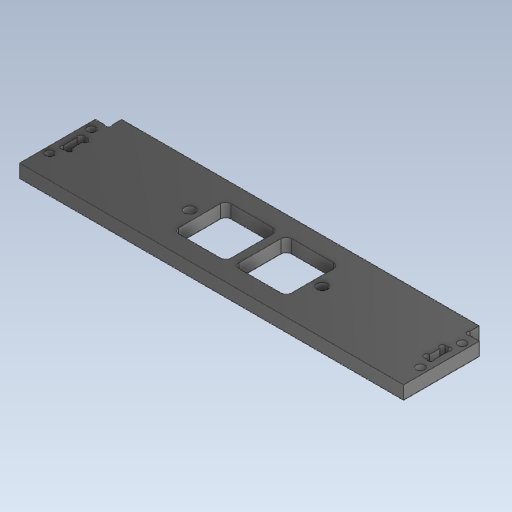
# Autodesk Inventor part: Cockpit_top_frame
Saved by Autodesk Inventor 2020.4 (Build 244396000, 396)
## iProperties
Created: 2022-01-28
Part Number: Cockpit_top_frame
Material: アセタール樹脂、黒
Document SubType Name: Modeling
Designer: Masato Kubotera
Density: 1.425 g/cm^3
Appearance: 滑らか - 黒
Description: POM T5
Author: Masato Kubotera
Autodesk Inventor part; units mm, degrees
ref_plane "YZ Plane" through (0, 0, 0) normal (1, 0, 0) x (0, 1, 0)
ref_plane "XZ Plane" through (0, 0, 0) normal (0, 1, 0) x (-1, 0, 0)
derived "Cockpit_side_frame.ipt"
sketch "スケッチ2" plane through (0, 0, 0) normal (0, 1, 0) x (-1, 0, 0)
  line L0 (-28.5, -22.5) -> (88.5, -22.5) construction
  line L1 (88.5, -22.5) -> (88.5, -138.5)
  line L2 (88.5, -96) -> (-28.5, -96) construction
  line L3 (-28.5, -96) -> (-28.5, -22.5) construction
  line L4 (-28.5, -22.5) -> (88.5, -96) construction
  line L5 (88.5, -22.5) -> (-28.5, -96) construction
  line L6 (38.5, -101) -> (38.5, -133.5)
  line L7 (43.5, -138.5) -> (88.5, -138.5)
  arc A0 (64.6349, -63.15) -> (63.15, -64.6349) centre (63.8925, -63.8925) ccw
  arc A1 (73.15, -65.2849) -> (71.6651, -63.8) centre (72.4075, -64.5425) ccw
  line L8 (65.3349, -63.8) -> (71.6651, -63.8)
  line L9 (64.6349, -63.15) -> (72.3651, -63.15)
  line L10 (63.9, -63.85) -> (73.1, -63.85) construction
  arc A2 (65.3349, -63.8) -> (63.85, -65.2849) centre (64.5925, -64.5425) ccw
  line L11 (63.2, -63.2) -> (73.8, -63.2) construction
  line L12 (73.15, -65.2849) -> (73.15, -76.2151)
  line L13 (73.8, -70.75) -> (63.2, -70.75) construction
  line L14 (73.85, -64.6349) -> (73.85, -76.8651)
  line L15 (73.1, -63.85) -> (73.1, -77.65) construction
  line L16 (63.85, -65.2849) -> (63.85, -76.2151)
  line L17 (73.8, -63.2) -> (73.8, -78.3) construction
  line L18 (63.15, -64.6349) -> (63.15, -76.8651)
  line L19 (68.5, -63.2) -> (68.5, -78.3) construction
  line L20 (63.9, -77.65) -> (63.9, -63.85) construction
  line L21 (73.1, -63.85) -> (63.9, -77.65) construction
  line L22 (73.8, -63.2) -> (63.2, -78.3) construction
  line L23 (63.2, -63.2) -> (73.8, -78.3) construction
  line L24 (63.2, -78.3) -> (63.2, -63.2) construction
  line L25 (63.9, -63.85) -> (73.1, -77.65) construction
  arc A3 (73.85, -64.6349) -> (72.3651, -63.15) centre (73.1075, -63.8925) ccw
  line L26 (73.1, -77.65) -> (63.9, -77.65) construction
  line L27 (73.8, -78.3) -> (63.2, -78.3) construction
  arc A4 (63.85, -76.2151) -> (65.3349, -77.7) centre (64.5925, -76.9575) ccw
  arc A5 (63.15, -76.8651) -> (64.6349, -78.35) centre (63.8925, -77.6075) ccw
  line L28 (65.3349, -77.7) -> (71.6651, -77.7)
  line L29 (64.6349, -78.35) -> (72.3651, -78.35)
  arc A6 (71.6651, -77.7) -> (73.15, -76.2151) centre (72.4075, -76.9575) ccw
  arc A7 (72.3651, -78.35) -> (73.85, -76.8651) centre (73.1075, -77.6075) ccw
  line L30 (-23.5, -22.5) -> (-28.5, -27.5)
  line L31 (-28.5, -59.25) -> (88.5, -59.25) construction
  line L32 (30, -22.5) -> (30, -96) construction
  line L33 (-23.5, -96) -> (-28.5, -91)
  line L34 (-28.5, -27.5) -> (-28.5, -91)
  line L35 (-20.5, -24.5) -> (-25.5, -24.5) construction
  line L36 (-25.5, -24.5) -> (-25.5, -94) construction
  line L37 (-25.5, -94) -> (-20.5, -94) construction
  line L38 (-20.5, -94) -> (-20.5, -24.5) construction
  line L39 (-20.5, -24.5) -> (-25.5, -94) construction
  line L40 (-25.5, -24.5) -> (-20.5, -94) construction
  line L41 (-25.55, -46.7) -> (-20.45, -46.7)
  line L42 (-20.45, -46.7) -> (-20.45, -71.8)
  line L43 (-20.45, -71.8) -> (-25.55, -71.8)
  line L44 (-25.55, -71.8) -> (-25.55, -46.7)
  line L45 (-25.55, -46.7) -> (-20.45, -71.8) construction
  line L46 (-20.45, -46.7) -> (-25.55, -71.8) construction
  line L47 (-25.5, -46.75) -> (-20.5, -46.75) construction
  line L48 (-25.5, -71.75) -> (-20.5, -71.75) construction
  line L49 (-23, -24.5) -> (-23, -94) construction
  circle A8 centre (-23, -35) radius 3
  circle A9 centre (-23, -35) radius 1.6
  arc A10 (-24.0651, -46.7) -> (-25.55, -48.1849) centre (-24.8075, -47.4425) ccw
  arc A11 (-20.45, -48.1849) -> (-21.9349, -46.7) centre (-21.1925, -47.4425) ccw
  arc A12 (-21.9349, -71.8) -> (-20.45, -70.3151) centre (-21.1925, -71.0575) ccw
  arc A13 (-25.55, -70.3151) -> (-24.0651, -71.8) centre (-24.8075, -71.0575) ccw
  circle A14 centre (-23, -83.5) radius 1.6
  circle A15 centre (-23, -83.5) radius 3
  line L50 (33.5, -96) -> (38.5, -101)
  line L51 (-23.5, -96) -> (33.5, -96)
  line L52 (81, -46.5) -> (-20.5, -46.5) construction
  line L53 (-20.5, -46.5) -> (-20.5, -41.5) construction
  line L54 (-20.5, -41.5) -> (81, -41.5) construction
  line L55 (81, -41.5) -> (81, -46.5) construction
  line L56 (81, -46.5) -> (-20.5, -41.5) construction
  line L57 (-20.5, -46.5) -> (81, -41.5) construction
  line L58 (-20.5, -44) -> (81, -44) construction
  line L59 (30.25, -41.5) -> (30.25, -46.5) construction
  line L60 (5.25, -41.5) -> (5.25, -46.5) construction
  line L61 (55.3, -41.45) -> (5.2, -41.45)
  line L62 (5.2, -41.45) -> (5.2, -46.55)
  line L63 (5.2, -46.55) -> (55.3, -46.55)
  line L64 (55.3, -46.55) -> (55.3, -41.45)
  line L65 (55.3, -41.45) -> (5.2, -46.55) construction
  line L66 (5.2, -41.45) -> (55.3, -46.55) construction
  arc A16 (6.6849, -41.45) -> (5.2, -42.9349) centre (5.9425, -42.1925) ccw
  circle A17 centre (-2.25, -44) radius 3
  circle A18 centre (-2.25, -44) radius 1.6
  line L67 (55.25, -41.5) -> (55.25, -46.5) construction
  arc A19 (55.3, -42.9349) -> (53.8151, -41.45) centre (54.5575, -42.1925) ccw
  circle A20 centre (62.75, -44) radius 3
  circle A21 centre (62.75, -44) radius 1.6
  arc A22 (5.2, -45.0651) -> (6.6849, -46.55) centre (5.9425, -45.8075) ccw
  arc A23 (53.8151, -46.55) -> (55.3, -45.0651) centre (54.5575, -45.8075) ccw
  line L68 (-20.5, -89) -> (81, -89) construction
  line L69 (81, -89) -> (81, -94) construction
  line L70 (81, -94) -> (-20.5, -94) construction
  line L71 (-20.5, -94) -> (-20.5, -89) construction
  line L72 (-20.5, -89) -> (81, -94) construction
  line L73 (81, -89) -> (-20.5, -94) construction
  line L74 (-20.5, -91.5) -> (81, -91.5) construction
  line L75 (30.25, -89) -> (30.25, -94) construction
  line L76 (55.3, -91.55) -> (5.2, -91.55)
  line L77 (5.2, -91.55) -> (5.2, -88.95)
  line L78 (5.2, -88.95) -> (55.3, -88.95)
  line L79 (55.3, -88.95) -> (55.3, -91.55)
  line L80 (55.3, -91.55) -> (5.2, -88.95) construction
  line L81 (5.2, -91.55) -> (55.3, -88.95) construction
  line L82 (5.25, -89) -> (5.25, -91.5) construction
  line L83 (55.25, -89) -> (55.25, -91.5) construction
  line L84 (5.25, -90.25) -> (55.25, -90.25) construction
  arc A24 (7.3, -88.95) -> (5.2, -88.95) centre (6.25, -88.95) ccw
  arc A25 (55.3, -88.95) -> (53.2, -88.95) centre (54.25, -88.95) ccw
  arc A26 (53.2, -91.55) -> (55.3, -91.55) centre (54.25, -91.55) ccw
  arc A27 (5.2, -91.55) -> (7.3, -91.55) centre (6.25, -91.55) ccw
  circle A28 centre (-2.5, -91.5) radius 3
  circle A29 centre (-2.5, -91.5) radius 1.6
  circle A30 centre (62.5, -91.5) radius 3 construction
  circle A31 centre (62.5, -91.5) radius 1.6 construction
  line L85 (-23.5, -22.5) -> (63.7651, -22.5)
  line L86 (65.25, -21.0151) -> (65.25, -17.5)
  line L87 (65.25, -17.5) -> (73.25, -17.5)
  line L88 (73.25, -17.5) -> (73.25, -21.0151)
  line L89 (81, -22.5) -> (81, -17.5)
  line L90 (88.5, -22.5) -> (88.5, -20)
  line L91 (81, -17.5) -> (86, -17.5)
  line L92 (86, -17.5) -> (88.5, -20)
  line L93 (69.25, -17.5) -> (69.25, -22.5) construction
  arc A32 (63.7651, -22.5) -> (65.25, -21.0151) centre (64.5075, -21.7575) ccw
  arc A33 (73.25, -21.0151) -> (74.7349, -22.5) centre (73.9925, -21.7575) ccw
  arc A34 (79.5151, -22.5) -> (81, -21.0151) centre (80.2575, -21.7575) ccw
  line L94 (-15.5, -89) -> (-15.5, -69) construction
  line L95 (-15.5, -69) -> (64.5, -69) construction
  line L96 (64.5, -69) -> (64.5, -89) construction
  line L97 (45.5, -84) -> (-16.5, -84)
  line L98 (-18.5, -82) -> (-18.5, -63.3955)
  line L99 (-16.5, -61.3955) -> (45.5, -61.3955)
  line L100 (47.5, -63.3955) -> (47.5, -82)
  line L101 (47.5, -84) -> (-18.5, -61.3955) construction
  line L102 (-18.5, -84) -> (47.5, -61.3955) construction
  arc A35 (-16.5, -61.3955) -> (-18.5, -63.3955) centre (-16.5, -63.3955) ccw
  arc A36 (-18.5, -82) -> (-16.5, -84) centre (-16.5, -82) ccw
  arc A37 (45.5, -84) -> (47.5, -82) centre (45.5, -82) ccw
  arc A38 (47.5, -63.3955) -> (45.5, -61.3955) centre (45.5, -63.3955) ccw
  line L103 (38.5, -133.5) -> (43.5, -138.5)
  line L104 (46, -131) -> (41, -131) construction
  line L105 (41, -131) -> (41, -96) construction
  line L106 (41, -96) -> (46, -96) construction
  line L107 (46, -96) -> (46, -131) construction
  line L108 (46, -131) -> (41, -96) construction
  line L109 (41, -131) -> (46, -96) construction
  line L110 (43.5, -96) -> (43.5, -131) construction
  line L111 (41, -113.5) -> (46, -113.5) construction
  line L112 (43.5, -107.5) -> (46, -107.5) construction
  line L113 (43.45, -107.45) -> (46.05, -107.45)
  line L114 (46.05, -107.45) -> (46.05, -119.55)
  line L115 (46.05, -119.55) -> (43.45, -119.55)
  line L116 (43.45, -119.55) -> (43.45, -107.45)
  line L117 (43.45, -107.45) -> (46.05, -119.55) construction
  line L118 (46.05, -107.45) -> (43.45, -119.55) construction
  arc A39 (46.05, -109.55) -> (46.05, -107.45) centre (46.05, -108.5) ccw
  arc A40 (44.9349, -107.45) -> (43.45, -108.9349) centre (44.1925, -108.1925) ccw
  arc A41 (46.05, -119.55) -> (46.05, -117.45) centre (46.05, -118.5) ccw
  line L119 (43.5, -119.5) -> (46, -119.5) construction
  arc A42 (43.45, -118.0651) -> (44.9349, -119.55) centre (44.1925, -118.8075) ccw
  line L120 (44.75, -107.5) -> (44.75, -119.5) construction
  circle A43 centre (43.5, -125.5) radius 3 construction
  circle A44 centre (43.5, -125.5) radius 1.6 construction
  circle A45 centre (43.5, -101.5) radius 3
  circle A46 centre (43.5, -101.5) radius 1.6
  circle A47 centre (-13.5, -55) radius 2
  line L121 (41, -131) -> (79.8645, -131) construction
  line L122 (79.8645, -131) -> (79.8645, -136) construction
  line L123 (79.8645, -136) -> (41, -136) construction
  line L124 (41, -136) -> (41, -131) construction
  line L125 (41, -131) -> (79.8645, -136) construction
  line L126 (79.8645, -131) -> (41, -136) construction
  line L127 (41, -133.5) -> (79.8645, -133.5) construction
  line L128 (60.4322, -131) -> (60.4322, -136) construction
  line L129 (60.4322, -133.5) -> (60.4322, -131) construction
  line L130 (52.8822, -130.95) -> (67.9822, -130.95)
  line L131 (67.9822, -130.95) -> (67.9822, -133.55)
  line L132 (67.9822, -133.55) -> (52.8822, -133.55)
  line L133 (52.8822, -133.55) -> (52.8822, -130.95)
  line L134 (52.8822, -130.95) -> (67.9822, -133.55) construction
  line L135 (67.9822, -130.95) -> (52.8822, -133.55) construction
  line L136 (52.9322, -131) -> (52.9322, -133.5) construction
  arc A48 (54.9822, -130.95) -> (52.8822, -130.95) centre (53.9322, -130.95) ccw
  arc A49 (52.8822, -132.0651) -> (54.3672, -133.55) centre (53.6247, -132.8075) ccw
  arc A50 (67.9822, -130.95) -> (65.8822, -130.95) centre (66.9322, -130.95) ccw
  arc A51 (66.4973, -133.55) -> (67.9822, -132.0651) centre (67.2398, -132.8075) ccw
  line L137 (67.9322, -131) -> (67.9322, -133.5) construction
  line L138 (52.9322, -132.25) -> (67.9322, -132.25) construction
  circle A52 centre (74.4322, -133.5) radius 1.6 construction
  circle A53 centre (74.4322, -133.5) radius 3 construction
  circle A54 centre (46.4322, -133.5) radius 3
  circle A55 centre (46.4322, -133.5) radius 1.6
  line L139 (50.5, -96.5) -> (79, -96.5)
  line L140 (81, -98.5) -> (81, -126.5)
  line L141 (79, -128.5) -> (50.5, -128.5)
  line L142 (48.5, -126.5) -> (48.5, -98.5)
  line L143 (48.5, -96.5) -> (81, -128.5) construction
  line L144 (81, -96.5) -> (48.5, -128.5) construction
  arc A56 (50.5, -96.5) -> (48.5, -98.5) centre (50.5, -98.5) ccw
  arc A57 (48.5, -126.5) -> (50.5, -128.5) centre (50.5, -126.5) ccw
  arc A58 (79, -128.5) -> (81, -126.5) centre (79, -126.5) ccw
  arc A59 (81, -98.5) -> (79, -96.5) centre (79, -98.5) ccw
  line L145 (81, -91.6746) -> (86, -91.6746) construction
  line L146 (86, -91.6746) -> (86, -136) construction
  line L147 (86, -136) -> (81, -136) construction
  line L148 (81, -136) -> (81, -91.6746) construction
  line L149 (81, -91.6746) -> (86, -136) construction
  line L150 (86, -91.6746) -> (81, -136) construction
  line L151 (83.5, -91.6746) -> (83.5, -136) construction
  circle A60 centre (83.5, -94.1746) radius 1.475
  circle A61 centre (83.5, -99.1746) radius 1.475
  circle A62 centre (83.5, -104.1746) radius 1.475
  circle A63 centre (83.5, -133.5) radius 1.6
  arc A64 (86, -91.6746) -> (81, -91.6746) centre (83.5, -133.5) ccw construction
  arc A65 (86.0112, -91.5751) -> (80.9888, -91.5751) centre (83.5, -133.5) ccw construction
  line L152 (88.5, -133.5) -> (83.5, -138.5)
  arc A66 (81, -131) -> (86, -136) centre (83.5, -133.5) ccw construction
  line L153 (86, -91.5) -> (81, -91.5) construction
  circle A67 centre (83.5, -133.5) radius 3
  line L154 (77.125, -22.5) -> (77.125, -27.147) construction
  line L155 (61.375, -22.5) -> (61.375, -27.147) construction
  line L156 (65.25, -22.5) -> (73.25, -22.5)
  line L157 (-18.5, -29.5) -> (-18.5, -34.7517)
  line L158 (-16.5, -36.7517) -> (45.5, -36.7517)
  line L159 (47.5, -34.7517) -> (47.5, -29.5)
  line L160 (45.5, -27.5) -> (-16.5, -27.5)
  arc A68 (-16.5, -27.5) -> (-18.5, -29.5) centre (-16.5, -29.5) ccw
  arc A69 (-18.5, -34.7517) -> (-16.5, -36.7517) centre (-16.5, -34.7517) ccw
  arc A70 (45.5, -36.7517) -> (47.5, -34.7517) centre (45.5, -34.7517) ccw
  arc A71 (47.5, -29.5) -> (45.5, -27.5) centre (45.5, -29.5) ccw
  line L161 (81, -66.9105) -> (86, -66.9105) construction
  line L162 (86, -66.9105) -> (86, -46.9105) construction
  line L163 (86, -46.9105) -> (81, -46.9105) construction
  line L164 (81, -46.9105) -> (81, -66.9105) construction
  line L165 (81, -66.9105) -> (86, -46.9105) construction
  line L166 (86, -66.9105) -> (81, -46.9105) construction
  line L167 (81, -22.5) -> (81, -28.5) construction
  line L168 (81, -28.5) -> (57.5, -28.5) construction
  line L169 (57.5, -28.5) -> (57.5, -22.5) construction
  line L170 (74.7349, -22.5) -> (79.5151, -22.5) construction
  line L171 (74.7349, -22.5) -> (79.5151, -22.5)
  point P0 (0, 0)
  point P1 (30, -59.25)
  point P2 (-25.7227, -96)
  point P3 (63.85, -63.8)
  point P4 (63.15, -63.15)
  point P5 (68.5, -70.75)
  point P6 (-23, -59.25)
  point P7 (30.25, -44)
  point P8 (30.25, -91.5)
  point P9 (30.25, -90.25)
  point P10 (30.25, -90.25)
  point P11 (52.5, -22)
  point P12 (14.5, -72.6978)
  point P13 (-18.5, -61)
  point P14 (47.5, -61)
  point P15 (43.5, -113.5)
  point P16 (44.75, -113.5)
  point P17 (60.4322, -132.25)
  point P18 (64.75, -112.5)
  point P19 (83.5, -113.8373)
  point P20 (-18.5, -36.7517)
  point P21 (47.5, -27.5)
  point P22 (-18.5, -27.5)
  point P23 (73.7349, -22.5)
  point P24 (72.25, -21.0151)
  point P25 (64.4973, -133.55)
  point P26 (63.8822, -130.95)
  point P27 (65.9822, -132.0651)
  point P28 (41.45, -118.0651)
  point P29 (44.05, -117.45)
  point P30 (42.9349, -119.55)
  point P31 (-26.05, -70.3151)
  point P32 (-22.4349, -46.7)
  point P33 (-20.95, -48.1849)
  point P34 (-20.95, -70.3151)
  point P35 (-22.4349, -71.8)
  point P36 (-24.5651, -71.8)
  point P37 (54.05, -59.5651)
  point P38 (52.5651, -61.05)
  point P39 (5.4349, -61.05)
  point P40 (3.95, -59.5651)
  point P41 (52.5651, -55.95)
  point P42 (54.05, -57.4349)
  point P43 (51.95, -88.45)
  point P44 (51.95, -91.05)
  point P45 (6.05, -91.05)
  point P46 (80.4349, -79.8)
  point P47 (78.95, -78.3151)
  point P48 (72.25, -22.5)
  point P49 (83.5, -56.9105)
  point P50 (69.25, -28.5)
  dimension "d1" = 22.5
  dimension "d2" = 5
  measures "d1" vertical distance of L1.start point (0, 0)
  measures "d2" vertical distance of L1.start L91.end
ref_plane "作業平面1" through (0, 0, -22.5) normal (0, 0, 1) x (1, 0, 0)
sketch "スケッチ3" plane through (0, 0, -22.5) normal (0, 0, 1) x (1, 0, 0)
  line L0 (-86, -140) -> (-52.5, -140)
  line L1 (-52.5, -140) -> (-52.5, 5)
  line L2 (-52.5, 5) -> (-86, 5)
  line L3 (-86, 5) -> (-86, -140)
  line L4 (-86, -140) -> (-52.5, 5) construction
  line L5 (-52.5, -140) -> (-86, 5) construction
  line L6 (-73.25, 2.5) -> (-65.25, 2.5) construction
  line L7 (-65.25, 2.5) -> (-65.25, 0) construction
  line L8 (-65.25, 0) -> (-73.25, 0) construction
  line L9 (-73.25, 0) -> (-73.25, 2.5) construction
  line L10 (-73.25, 2.5) -> (-65.25, 0) construction
  line L11 (-65.25, 2.5) -> (-73.25, 0) construction
  line L12 (-81.05, 5) -> (-81.05, 0)
  line L13 (-81.05, 0) -> (-86, 0)
  arc A0 (-82.5349, 0) -> (-81.05, 1.4849) centre (-81.7925, 0.7425) ccw
  line L14 (-73.3, 2.55) -> (-65.2, 2.55)
  line L15 (-65.2, 2.55) -> (-65.2, -0.05)
  line L16 (-65.2, -0.05) -> (-73.3, -0.05)
  line L17 (-73.3, -0.05) -> (-73.3, 2.55)
  line L18 (-73.3, 2.55) -> (-65.2, -0.05) construction
  line L19 (-65.2, 2.55) -> (-73.3, -0.05) construction
  line L20 (-73.25, 1.25) -> (-65.25, 1.25) construction
  line L21 (-69.25, 2.5) -> (-69.25, 0) construction
  arc A1 (-71.8151, 2.55) -> (-73.3, 1.0651) centre (-72.5575, 1.8075) ccw
  arc A2 (-73.3, -0.05) -> (-71.2, -0.05) centre (-72.25, -0.05) ccw
  arc A3 (-65.2, 1.0651) -> (-66.6849, 2.55) centre (-65.9425, 1.8075) ccw
  arc A4 (-67.3, -0.05) -> (-65.2, -0.05) centre (-66.25, -0.05) ccw
  line L22 (-59.9, -65.42) -> (-78.6, -65.42) construction
  line L23 (-78.6, -65.42) -> (-78.6, -46.72) construction
  line L24 (-78.6, -46.72) -> (-59.9, -46.72) construction
  line L25 (-59.9, -46.72) -> (-59.9, -65.42) construction
  line L26 (-59.9, -65.42) -> (-78.6, -46.72) construction
  line L27 (-78.6, -65.42) -> (-59.9, -46.72) construction
  line L28 (-69.25, -56.07) -> (-69.25, -78.93) construction
  line L29 (-61.3142, -46.1342) -> (-77.1858, -46.1342)
  line L30 (-79.1858, -48.1342) -> (-79.1858, -64.0058)
  line L31 (-77.1858, -66.0058) -> (-61.3142, -66.0058)
  line L32 (-59.3142, -64.0058) -> (-59.3142, -48.1342)
  line L33 (-59.3142, -46.1342) -> (-79.1858, -66.0058) construction
  line L34 (-79.1858, -46.1342) -> (-59.3142, -66.0058) construction
  arc A5 (-59.3142, -48.1342) -> (-61.3142, -46.1342) centre (-61.3142, -48.1342) ccw
  arc A6 (-77.1858, -46.1342) -> (-79.1858, -48.1342) centre (-77.1858, -48.1342) ccw
  arc A7 (-79.1858, -64.0058) -> (-77.1858, -66.0058) centre (-77.1858, -64.0058) ccw
  arc A8 (-61.3142, -66.0058) -> (-59.3142, -64.0058) centre (-61.3142, -64.0058) ccw
  line L35 (-86, -67.5) -> (-52.5, -67.5)
  circle A9 centre (-77.125, 2.5) radius 1.6
  circle A10 centre (-61.375, 2.5) radius 1.6
  line L36 (-80.5, -96.5) -> (-58, -96.5) construction
  line L37 (-58, -96.5) -> (-58, -38.5) construction
  line L38 (-58, -38.5) -> (-80.5, -38.5) construction
  line L39 (-80.5, -38.5) -> (-80.5, -96.5) construction
  line L40 (-80.5, -96.5) -> (-58, -38.5) construction
  line L41 (-58, -96.5) -> (-80.5, -38.5) construction
  line L42 (-78.1, -47.22) -> (-60.4, -47.22) construction
  line L43 (-60.4, -47.22) -> (-60.4, -64.92) construction
  line L44 (-60.4, -64.92) -> (-78.1, -64.92) construction
  line L45 (-78.1, -64.92) -> (-78.1, -47.22) construction
  line L46 (-78.1, -47.22) -> (-60.4, -64.92) construction
  line L47 (-60.4, -47.22) -> (-78.1, -64.92) construction
  circle A11 centre (-69.25, -42.5) radius 1.6 construction
  circle A12 centre (-69.25, -42.5) radius 2
  line L48 (-78.1, -87.78) -> (-60.4, -87.78) construction
  line L49 (-60.4, -87.78) -> (-60.4, -70.08) construction
  line L50 (-60.4, -70.08) -> (-78.1, -70.08) construction
  line L51 (-78.1, -70.08) -> (-78.1, -87.78) construction
  circle A13 centre (-69.25, -92.5) radius 1.6 construction
  circle A14 centre (-69.25, -92.5) radius 2
  circle A15 centre (-69.25, -42.5) radius 3.5 construction
  point P0 (0, 0)
  point P1 (-69.25, -67.5)
  point P2 (-52.5, 0)
  point P3 (-69.25, 1.25)
  point P4 (-81, 0)
  point P5 (-81, 0)
  point P6 (-81, 0)
  point P7 (-69.25, -67.5)
  point P8 (-68.25, -67.5)
  point P9 (-69.25, -67.5)
  point P10 (-67.3, -0.05)
  point P11 (-66.6849, 2.55)
  point P12 (-65.2, 1.0651)
  point P13 (-77.125, 0)
  point P14 (-77.125, 0)
  point P15 (-61.375, 0)
  point P16 (-61.375, 0)
  point P17 (-61.375, 0)
  point P18 (-69.25, -67.5)
  dimension "d4" = 5
  dimension "d5" = 145
  dimension "d6" = 2.5
  dimension "d7" = 0.05
  dimension "d8" = 1.05
  dimension "d9" = 0.05
  dimension "d10" = 0.05
  dimension "d11" = 1.05
  dimension "d12" = 1.05
  dimension "d15" = 22.86
  dimension "d16" = 2
  dimension "d24" = 3.2
  dimension "d25" = 15.75
  dimension "d26" = 15.75
  dimension "d27" = 22.5
  dimension "d28" = 58
  dimension "d29" = 17.7
  dimension "d30" = 17.7
  dimension "d31" = 0.5
  dimension "d32" = 0.5
  dimension "d33" = 3.2
  dimension "d34" = 4
  dimension "d36" = 7
  dimension "d37" = 50
  constraints: 104 end point, 25 midpoint, 22 point on circle, 21 point on line, 16 centre point, 12 parallel, 12 symmetric about line, 8 perpendicular, 8 tangent, 7 horizontal, 4 coincident, 3 equal radius, 2 vertical, 5 other
  measures "d4" distance of L2.end L13.end
  measures "d5" distance of L0.end L1.end
  measures "d6" distance of L8.end L6.start
  measures "d7" distance of L12.end point (-81, 0)
  measures "d8" radius of A0
  measures "d9" horizontal distance of L14.start L6.start
  measures "d10" horizontal distance of L14.start L6.start
  measures "d11" radius of A1
  measures "d12" radius of A2
  measures "d15" distance of L28.start L28.end
  measures "d16" radius of A5
  measures "d24" diameter of A9
  measures "d25" distance of point (-77.125, 0) point (-61.375, 0)
  measures "d26" distance of A10.centre A9.centre
  measures "d27" distance of L38.end L37.end
  measures "d28" distance of L37.end L36.end
  measures "d29" distance of L43.end L44.end
  measures "d30" distance of L42.end L43.end
  measures "d31" distance between parallel lines of L25 L43
  measures "d32" distance between parallel lines of L24 L42
  measures "d33" diameter of A11
  measures "d34" diameter of A12
  measures "d36" diameter of A15
  measures "d37" distance of A14.centre A12.centre
extrude "押し出し1" add sketch "スケッチ3" along normal blind 5 contours L3 L13 A0 L12 L2 L1 L35
mirror "ミラー1" about plane through (-86, -67.5, -22.5) normal (0, -1, 0)
equation "\"d9\" = d7"
equation "\"d10\" = d9"
equation "\"d12\" = d11"
equation "\"d26\" = d25"
equation "\"d29\" = d30"
equation "\"d31\" = d32"
equation "\"d3\" = -d1"
